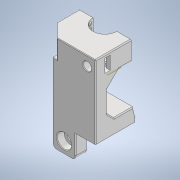
# Autodesk Inventor part: Left Cable Guide
Saved by Autodesk Inventor 2020 (Build 240168000, 168)
## iProperties
Created: 2019-11-15
Part Number: Left Cable Guide
Material: Generic
Document SubType Name: Modeling
Designer: pepd9
Density: 1 g/cm^3
Appearance: Default
Author: pepd9
Autodesk Inventor part; units mm, degrees
ref_plane "YZ Plane" through (0, 0, 0) normal (1, 0, 0) x (0, 1, 0)
ref_plane "XZ Plane" through (0, 0, 0) normal (0, 1, 0) x (-1, 0, 0)
ref_plane "XY Plane" through (0, 0, 0) normal (0, 0, 1) x (1, 0, 0)
sketch "Sketch1" plane through (0, 0, 0) normal (0, 0, 1) x (1, 0, 0)
  circle A0 centre (1.7413, 0) radius 1.7 projected
  arc A1 (4.7413, -5) -> (6.7413, -3) centre (4.7413, -3) ccw projected
  line L0 (6.7413, 5) -> (6.7413, -3) projected
  line L1 (-3.2587, 5) -> (6.7413, 5) projected
  line L2 (-3.2587, -3) -> (-3.2587, 5) projected
  arc A2 (-3.2587, -3) -> (-1.2587, -5) centre (-1.2587, -3) ccw projected
  line L3 (4.7413, -5) -> (-1.2587, -5) projected
  line L4 (-3.0587, 4.8) -> (6.5413, 4.8)
  line L5 (6.5413, 5) -> (6.5413, -3)
  arc A3 (4.7413, -4.8) -> (6.5413, -3) centre (4.7413, -3) ccw
  line L6 (4.7413, -4.8) -> (-1.2587, -4.8)
  arc A4 (-3.0587, -3) -> (-1.2587, -4.8) centre (-1.2587, -3) ccw
  line L7 (-3.0587, -3) -> (-3.0587, 5)
  dimension "d3" = 0.2
  constraints: 8 end point, 4 point on circle, 4 point on line, 2 centre point, 2 other
  measures "d3" distance between parallel lines of L2 L7
ref_plane "Work Plane1" through (-7.7587, -45, 5) normal (0, 0, 1) x (1, 0, 0)
extrude "Extrusion1" add sketch "Sketch1" along normal blind 4.9 contours L5 L4 L7 L1 | L5 A3 L6 A4 L7 L4
sketch "Sketch2" plane through (-4.8, 5, 4.9) normal (0, 0, 1) x (1, 0, 0)
  circle A0 centre (6.5413, -5) radius 1.7 projected
hole "Hole1" at (1.7413, 0, 4.9) direction (0, 0, -1) diameter 3.4 end through all counterbore diameter 6 counterbore depth 3 clearance for "Socket Head Cap Screw" size "M3" standard "Ansi Metric M Profile"
sketch "Sketch3" plane through (-3.0587, 5, 0) normal (0, 1, 0) x (1, 0, 0)
  line L0 (0, -4.9) -> (1.8, -4.9) projected
  line L1 (0, -4.9) -> (18, -4.9)
  line L2 (18, -4.9) -> (18, 12)
  line L3 (18, 12) -> (0, 12)
  line L4 (0, 12) -> (0, -4.9)
  line L5 (57.3, 12) -> (-0.7, 12) projected
  point P0 (3.0587, 0)
  point P1 (1.8, -4.9)
  dimension "d13" = 18
  constraints: 8 end point, 2 parallel, 1 horizontal, 1 perpendicular, 1 point on line
  measures "d13" distance of L3.end L2.end
extrude "Extrusion2" add sketch "Sketch3" along normal blind 6
sketch "Sketch4" plane through (-3.0587, 11, 0) normal (0, 1, 0) x (1, 0, 0)
  line L0 (0, 12) -> (0, -4.9) projected
  line L1 (0, -4.9) -> (18, -4.9)
  line L2 (18, -4.9) -> (18, 0.1)
  line L3 (18, 0.1) -> (0, 0.1)
  line L4 (0, 0.1) -> (0, -4.9)
  point P0 (3.0587, 0)
  point P1 (0, 0.1)
  dimension "d17" = 5
  constraints: 8 end point, 2 parallel, 1 horizontal, 1 perpendicular, 1 point on line
  measures "d17" distance of L2.end L1.end
extrude "Extrusion3" add sketch "Sketch4" along normal blind 25
sketch "Sketch5" plane through (-3.0587, 36, 0) normal (0, 1, 0) x (1, 0, 0)
  line L0 (0, 0.1) -> (0, -4.9) projected
  line L1 (0, -4.9) -> (18, -4.9) projected
  line L2 (18, -4.9) -> (18, 0.1) projected
  line L3 (18, 0.1) -> (0, 0.1) projected
  circle A0 centre (7, 10.1) radius 5
  line L4 (18, 0.1) -> (0, 0.1) projected
  line L5 (18, 0.1) -> (0, 0.1)
  line L6 (0, 0.1) -> (0, 10.1)
  line L7 (0, 10.1) -> (18, 10.1)
  line L8 (18, 10.1) -> (18, 0.1)
  point P0 (3.0587, 0)
  point P1 (12, 10.1)
  point P2 (7, 0.1)
  point P3 (2, 10.1)
  dimension "d20" = 10
  dimension "d21" = 7
  dimension "d22" = 10
  dimension "d23" = 18
  dimension "d24" = 10
  constraints: 8 end point, 2 parallel, 1 centre point, 1 horizontal, 1 perpendicular
  measures "d20" diameter of A0
  measures "d21" distance from line of L0 A0.centre
  measures "d22" distance from line of L3 A0.centre
  measures "d23" distance of L6.end L7.end
  measures "d24" distance between parallel lines of L3 L7
extrude "Extrusion4" add sketch "Sketch5" against normal blind 8 contours L6 L7 A0 L8 L3
ref_plane "Work Plane2" through (-3.0587, 28.5, 0) normal (0, -1, 0) x (1, 0, 0)
sketch "Sketch6" plane through (-3.0587, 28.5, 0) normal (0, -1, 0) x (1, 0, 0)
  arc A0 (12, -10.1) -> (2, -10.1) centre (7, -10.1) ccw projected
  arc A1 (11.5, -10.1) -> (2.5, -10.1) centre (7, -10.1) ccw
  line L0 (12, -10.1) -> (11.5, -10.1)
  line L1 (11.8547, -8.9034) -> (11.3692, -9.0231)
  line L2 (11.4273, -7.7764) -> (10.9846, -8.0087)
  line L3 (10.7426, -6.7844) -> (10.3683, -7.1159)
  line L4 (9.8403, -5.9851) -> (9.5563, -6.3966)
  line L5 (8.773, -5.4249) -> (8.5957, -5.8924)
  line L6 (7.6027, -5.1365) -> (7.5424, -5.6328)
  line L7 (6.3973, -5.1365) -> (6.4576, -5.6328)
  line L8 (5.227, -5.4249) -> (5.4043, -5.8924)
  line L9 (4.1597, -5.9851) -> (4.4437, -6.3966)
  line L10 (3.2574, -6.7844) -> (3.6317, -7.1159)
  line L11 (2.5727, -7.7764) -> (3.0154, -8.0087)
  line L12 (2.1453, -8.9034) -> (2.6308, -9.0231)
  line L13 (2, -10.1) -> (2.5, -10.1)
  point P0 (3.0587, 0)
  point P1 (2.1453, -8.9034)
  point P2 (2.6308, -9.0231)
  point P3 (3.0154, -8.0087)
  point P4 (2.5727, -7.7764)
  point P5 (3.6317, -7.1159)
  point P6 (4.1597, -5.9851)
  point P7 (5.4043, -5.8924)
  point P8 (6.4576, -5.6328)
  point P9 (7.5424, -5.6328)
  point P10 (8.5957, -5.8924)
  point P11 (9.8403, -5.9851)
  point P12 (9.5563, -6.3966)
  point P13 (10.3683, -7.1159)
  point P14 (11.4273, -7.7764)
  point P15 (10.9846, -8.0087)
  point P16 (11.3692, -9.0231)
  dimension "d28" = 0.5
  dimension "d31" = 180
  constraints: 28 end point, 2 point on circle, 1 centre point, 1 horizontal, 40 other
  measures "d28" radial gap between concentric circles of A0 A1
extrude "Extrusion5" add sketch "Sketch6" against normal blind 0.75 contours L1 A1 L2 A0 | L3 A1 L4 A0 | L5 A1 L6 A0 | L7 A1 L8 A0 | L9 A1 L10 A0 | L11 A1 L12 A0
pattern_linear "Rectangular Pattern1" count 4 spacing 2 along (0, 1, 0) of "Extrusion5"
sketch "Sketch7" plane through (14.9413, 36, -10.1) normal (0, 0, -1) x (-1, 0, 0)
  line L0 (0, 0) -> (6, 0) projected
  line L1 (0, 0) -> (0, -8) projected
  line L2 (6, -8) -> (0, -8) projected
  line L3 (6, 0) -> (6, -8) projected
  point P0 (14.9413, -36)
  point P1 (3.5, -4)
  dimension "d45" = 4
  dimension "d46" = 2.5
  measures "d45" distance from line of L0 point (3.5, -4)
  measures "d46" distance from line of L3 point (3.5, -4)
hole "Hole2" at (11.4413, 32, -10.1) direction (0, 0, 1) diameter 3.4 end through all
chamfer "Chamfer1" distance 5 angle 45 1 edges at (5.9413, 28, -0.1)
chamfer "Chamfer2" distance 3 angle 45 1 edges at (5.9413, 11, -0.1)
chamfer "Chamfer3" distance 4 distance2 1 1 edges at (5.9413, 11, -12) measured on face at (5.9413, 10.5, -12)
sketch "Sketch8" plane through (14.9413, 5, 4.9) normal (1, 0, 0) x (0, 0, -1)
  line L0 (0, 25.3) -> (0, 28.7) projected
  line L1 (15, 28.7) -> (15, 25.3) projected
  line L2 (0, 25.3) -> (0, 28.7) projected
  line L3 (0, 27) -> (15, 27)
  line L4 (15, 28.7) -> (15, 25.3) projected
  line L5 (4, 24.2) -> (6.25, 24.2)
  line L6 (6.25, 24.2) -> (6.25, 29.8)
  line L7 (6.25, 29.8) -> (4, 29.8)
  line L8 (4, 29.8) -> (4, 24.2)
  line L9 (4, 24.2) -> (6.25, 29.8) construction
  line L10 (6.25, 24.2) -> (4, 29.8) construction
  point P0 (4.9, -5)
  point P1 (5.125, 27)
  dimension "d56" = 2.25
  dimension "d57" = 5.6
  dimension "d58" = 4
  constraints: 14 end point, 4 midpoint, 2 parallel, 1 horizontal, 1 perpendicular, 1 point on line
  measures "d56" distance of L7.end L6.end
  measures "d57" distance of L6.end L5.end
  measures "d58" distance between parallel lines of L0 L8
extrude "Extrusion6" cut sketch "Sketch8" against normal blind 6.25
sketch "Sketch10" plane through (-3.0587, 36, 0) normal (0, 1, 0) x (1, 0, 0)
  line L0 (2, 10.1) -> (0, 10.1) projected
  line L1 (2, 10.1) -> (-4, 10.1)
  line L2 (-4, 10.1) -> (-4, -4.9)
  line L3 (-4, -4.9) -> (2, -4.9)
  line L4 (2, -4.9) -> (2, 10.1)
  point P0 (3.0587, 0)
  dimension "d69" = 6
  dimension "d70" = 15
  constraints: 8 end point, 2 parallel, 1 horizontal, 1 perpendicular
  measures "d69" distance of L3.end L2.end
  measures "d70" distance of L2.end L1.end
extrude "Extrusion8" add sketch "Sketch10" against normal up to surface (8 mm away)
sketch "Sketch11" plane through (-1.0587, 28, -10.1) normal (0, 0, -1) x (-1, 0, 0)
  line L0 (0, 8) -> (6, 8) projected
  line L1 (0, 8) -> (0, 0) projected
  line L2 (6, 0) -> (0, 0) projected
  line L3 (6, 8) -> (6, 0) projected
  point P0 (-1.0587, -28)
  point P1 (2.5, 4)
  dimension "d73" = 2.5
  dimension "d74" = 4
  measures "d73" distance from line of L1 point (2.5, 4)
  measures "d74" distance from line of L0 point (2.5, 4)
hole "Hole3" at (-3.5587, 32, -10.1) direction (0, 0, 1) diameter 3.4 end through all clearance for "Socket Head Cap Screw" size "M3" standard "Ansi Metric M Profile"
sketch "Sketch12" plane through (-3.0587, 36, 0) normal (0, 1, 0) x (1, 0, 0)
  line L0 (0, -4.9) -> (-4, -4.9) projected
  line L1 (-4, -4.9) -> (2, -4.9)
  line L2 (2, -4.9) -> (2, -4.89)
  line L3 (2, -4.89) -> (-4, -4.89)
  line L4 (-4, -4.89) -> (-4, -4.9)
  point P0 (3.0587, 0)
  point P1 (0, -4.9)
  point P2 (0, -4.9)
  dimension "d82" = 6
  dimension "d83" = 0.01
  constraints: 8 end point, 2 parallel, 1 horizontal, 1 perpendicular
  measures "d82" distance of L3.end L2.end
  measures "d83" distance of L2.end L1.end
extrude "Extrusion9" cut sketch "Sketch12" against normal blind 8
chamfer "Chamfer5" distance 6 angle 45 1 edges at (-7.0587, 32, 4.89)
sketch "Sketch13" plane through (-7.0587, 28, -10.1) normal (-1, 0, 0) x (0, 0, 1)
  line L0 (0, 2.3) -> (0, 5.7) projected
  circle A0 centre (12.49, 4) radius 1.7 projected
  line L1 (0, 8) -> (0, 0) projected
  line L2 (0, 4) -> (12.49, 4)
  line L3 (6, 1.2) -> (8.25, 1.2)
  line L4 (8.25, 1.2) -> (8.25, 6.8)
  line L5 (8.25, 6.8) -> (6, 6.8)
  line L6 (6, 6.8) -> (6, 1.2)
  line L7 (6, 1.2) -> (8.25, 6.8) construction
  line L8 (8.25, 1.2) -> (6, 6.8) construction
  point P0 (10.1, -28)
  point P1 (7.125, 4)
  dimension "d89" = 2.25
  dimension "d90" = 5.6
  dimension "d91" = 6
  constraints: 14 end point, 3 midpoint, 2 horizontal, 2 parallel, 1 perpendicular, 1 point on line
  measures "d89" distance of L5.end L4.end
  measures "d90" distance of L4.end L3.end
  measures "d91" distance between parallel lines of L1 L6
extrude "Extrusion10" cut sketch "Sketch13" against normal blind 6.5 contours L6 L5 L4 L2 | L2 L4 L3 L6
sketch "Sketch14" plane through (-7.0587, 29.2, -4.1) normal (0, 0, 1) x (1, 0, 0)
  line L0 (1.8, -0.5872) -> (5.2, -0.5872)
  line L1 (5.2, -0.5872) -> (5.2, 6.1872)
  line L2 (5.2, 6.1872) -> (1.8, 6.1872)
  line L3 (1.8, 6.1872) -> (1.8, -0.5872)
  circle A0 centre (3.5, 2.8) radius 1.7 projected
  line L4 (1.8, -0.5872) -> (5.2, 6.1872) construction
  line L5 (5.2, -0.5872) -> (1.8, 6.1872) construction
  circle A1 centre (3.5, 2.8) radius 1.7 projected
  line L6 (0, 0) -> (0, 5.6) projected
  line L7 (0, 0) -> (6.5, 0) projected
  line L8 (6.5, 0) -> (6.5, 5.6) projected
  line L9 (0, 5.6) -> (6.5, 5.6) projected
  point P0 (7.0587, -29.2)
  point P1 (5.2, 5.6)
  point P2 (1.8, 5.6)
  point P3 (1.8, 2.8)
  point P4 (5.2, 2.8)
  point P5 (1.8, 0)
  point P6 (5.2, 0)
  dimension "d94" = 3.4
  constraints: 12 end point, 2 midpoint, 2 parallel, 1 horizontal, 1 perpendicular
  measures "d94" distance of L2.end L1.end
extrude "Extrusion11" cut sketch "Sketch14" against normal blind 0.5 contours L3 A0 L1 L7 | L3 L9 L1 A0
sketch "Sketch15" plane through (-7.0587, 29.2, -4.6) normal (0, 0, 1) x (1, 0, 0)
  line L0 (5.2, 2.8) -> (5.2, 0) projected
  arc A0 (1.8, 2.8) -> (5.2, 2.8) centre (3.5, 2.8) ccw projected
  line L1 (1.8, 0) -> (1.8, 2.8) projected
  line L2 (5.2, 0) -> (1.8, 0) projected
  line L3 (1.8, 5.6) -> (5.2, 5.6) projected
  line L4 (1.8, 2.8) -> (1.8, 5.6) projected
  arc A1 (5.2, 2.8) -> (1.8, 2.8) centre (3.5, 2.8) ccw projected
  line L5 (5.2, 5.6) -> (5.2, 2.8) projected
  line L6 (5.2, 1.1) -> (1.8, 1.1)
  line L7 (1.8, 1.1) -> (1.8, 4.5)
  line L8 (1.8, 4.5) -> (5.2, 4.5)
  line L9 (5.2, 4.5) -> (5.2, 1.1)
  line L10 (5.2, 1.1) -> (1.8, 4.5) construction
  line L11 (1.8, 1.1) -> (5.2, 4.5) construction
  point P0 (7.0587, -29.2)
  point P1 (1.8, 4.5)
  point P2 (1.8, 2.8)
  point P3 (1.8, 1.1)
  point P4 (5.2, 1.1)
  point P5 (5.2, 2.8)
  point P6 (5.2, 4.5)
  dimension "d97" = 3.4
  dimension "d98" = 3.4
  constraints: 12 end point, 2 midpoint, 2 parallel, 1 horizontal, 1 perpendicular
  measures "d97" distance of L7.end L8.end
  measures "d98" distance of L6.end L7.end
extrude "Extrusion12" cut sketch "Sketch15" against normal blind 0.5 contours L0 L6 A0 | A0 A1 | A1 L8 L5 | L6 L1 A0 | A1 L4 L8
sketch "Sketch16" plane through (14.9413, 29.2, -1.35) normal (0, 0, 1) x (1, 0, 0)
  circle A0 centre (-3.5, 2.8) radius 1.7 projected
  line L0 (0, 5.6) -> (0, 0) projected
  line L1 (0, 5.6) -> (-6.25, 5.6) projected
  line L2 (-6.25, 5.6) -> (-6.25, 0) projected
  line L3 (0, 0) -> (-6.25, 0) projected
  line L4 (-5.2, -0.5689) -> (-1.8, -0.5689)
  line L5 (-1.8, -0.5689) -> (-1.8, 6.1689)
  line L6 (-1.8, 6.1689) -> (-5.2, 6.1689)
  line L7 (-5.2, 6.1689) -> (-5.2, -0.5689)
  circle A1 centre (-3.5, 2.8) radius 1.7 projected
  line L8 (-5.2, -0.5689) -> (-1.8, 6.1689) construction
  line L9 (-1.8, -0.5689) -> (-5.2, 6.1689) construction
  point P0 (-14.9413, -29.2)
  point P1 (-5.2, 5.6)
  point P2 (-5.2, 2.8)
  point P3 (-1.8, 2.8)
  point P4 (-1.8, 5.6)
  point P5 (-5.2, 0)
  point P6 (-1.8, 0)
  dimension "d101" = 3.4
  constraints: 12 end point, 2 midpoint, 2 parallel, 1 horizontal, 1 perpendicular
  measures "d101" distance of L6.end L5.end
extrude "Extrusion13" cut sketch "Sketch16" against normal blind 0.5 contours L5 L3 L7 A0 | A0 L7 L1 L5
sketch "Sketch17" plane through (14.9413, 29.2, -1.85) normal (0, 0, 1) x (1, 0, 0)
  line L0 (-1.8, 2.8) -> (-1.8, 0) projected
  arc A0 (-5.2, 2.8) -> (-1.8, 2.8) centre (-3.5, 2.8) ccw projected
  line L1 (-5.2, 0) -> (-5.2, 2.8) projected
  line L2 (-1.8, 0) -> (-5.2, 0) projected
  line L3 (-1.8, 5.6) -> (-1.8, 2.8) projected
  line L4 (-5.2, 5.6) -> (-1.8, 5.6) projected
  line L5 (-5.2, 2.8) -> (-5.2, 5.6) projected
  arc A1 (-1.8, 2.8) -> (-5.2, 2.8) centre (-3.5, 2.8) ccw projected
  line L6 (-5.2, 1.1) -> (-1.8, 1.1)
  line L7 (-1.8, 1.1) -> (-1.8, 4.5)
  line L8 (-1.8, 4.5) -> (-5.2, 4.5)
  line L9 (-5.2, 4.5) -> (-5.2, 1.1)
  line L10 (-5.2, 1.1) -> (-1.8, 4.5) construction
  line L11 (-1.8, 1.1) -> (-5.2, 4.5) construction
  point P0 (-14.9413, -29.2)
  point P1 (-1.8, 4.5)
  point P2 (-5.2, 4.5)
  point P3 (-5.2, 2.8)
  point P4 (-5.2, 1.1)
  point P5 (-1.8, 1.1)
  point P6 (-1.8, 2.8)
  dimension "d104" = 3.4
  dimension "d105" = 3.4
  constraints: 12 end point, 2 midpoint, 2 parallel, 1 horizontal, 1 perpendicular
  measures "d104" distance of L8.end L7.end
  measures "d105" distance of L7.end L6.end
extrude "Extrusion14" cut sketch "Sketch17" against normal blind 0.5 contours L0 L6 A0 | A1 L8 L3 | A0 A1 | L6 L1 A0 | A1 L5 L8
chamfer "Chamfer6" distance 0.25 angle 45 11 edges at (1.7413, -4.8, 4.9) (6.0141, -4.2728, 4.9) (6.5413, 1, 4.9) (-2.5315, -4.2728, 4.9) (-3.0587, 12.5, 4.9) (10.7413, 5, 4.9) (14.9413, 20.5, 4.9) (6.9413, 36, 4.9) (-2.0587, 28, 4.9) (1.7413, 3, 4.9) (11.4413, 30.3, 4.9)
chamfer "Chamfer7" distance 0.25 angle 45 7 edges at (-3.0587, 5, -6) (14.9413, 5, -3.675) (-3.0587, 1, 0) (-2.5315, -4.2728, 0) (1.7413, -4.8, 0) (6.0141, -4.2728, 0) (6.5413, 1, 0)
fillet "Fillet1" radius 0.4 16 edges at (-3.0587, 11, -7.05) (-3.0587, 12.5, -1.6) (-3.0587, 18.5001, -0.1) (-3.0587, 25.5001, -2.5999) (-3.0587, 9, -11.5) (-3.0587, 6.125, -12) (14.9413, 6.125, -12) (14.9413, 9, -11.5) (14.9413, 11, -7.05) (14.9413, 12.5, -1.6) (14.9413, 18.5, -0.1) (14.9413, 25.5, -2.5999) (14.9413, 28, -7.5999) (-7.0587, 28, -5.605) (-7.0587, 36, -5.605) (14.9413, 36, -2.725)
chamfer "Chamfer8" distance 0.25 angle 45 2 edges at (-3.5587, 30.3, -10.1) (11.4413, 30.3, -10.1)
body "Solid1"
